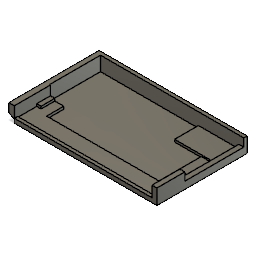
EZ Flash Shell v1 (Autodesk Fusion 360 design; units mm, degrees)
Autodesk Fusion 360 part; units mm, degrees
sketch "Sketch1" plane through (0, 0, 0) normal (0, 1, 0) x (1, 0, 0)
  line L0 (0, 0) -> (53.1, 0)
  line L1 (53.1, 0) -> (53.1, 32)
  line L2 (53.1, 32) -> (0, 32)
  line L3 (0, 32) -> (0, 0)
  line L4 (26.55, 0) -> (26.55, -1.25)
  line L5 (26.55, -1.25) -> (26.55, 33.35)
  line L6 (26.55, 33.35) -> (55, 33.35)
  line L7 (55, 33.35) -> (-1.9, 33.35)
  line L8 (-1.9, 33.35) -> (-1.9, -1.25)
  line L9 (-1.9, -1.25) -> (55, -1.25)
  line L10 (55, -1.25) -> (55, 33.35)
  dimension "d1" = 53.1
  dimension "d2" = 32
  dimension "d3" = 1.25
  dimension "d4" = 34.6
  dimension "d5" = 28.45
  dimension "d6" = 56.9
  dimension "d7" = 34.6
  constraint horizontal L0
  constraint vertical L1
  constraint horizontal L2
  constraint vertical L3
  constraint coincident L0.start L3.end
  constraint midpoint L0 L4.start
  constraint vertical L4
  constraint parallel L4 L5
  constraint perpendicular L5 L6
  constraint horizontal L7
  constraint vertical L8
  constraint horizontal L9
  constraint vertical L10
  measures "d1" distance of L0.start L0.end
  measures "d2" distance of L0.start L2.end
  measures "d3" distance of L4.start L4.end
  measures "d4" distance of L4.end L5.end
  measures "d5" distance of L5.end L6.end
  measures "d6" distance of L6.end L7.end
  measures "d7" distance of L6.end L9.end
extrude "Extrude1" add sketch "Sketch1" along normal blind 1.5
sketch "Sketch2" plane through (0, 1.5, 0) normal (0, 1, 0) x (-1, 0, 0)
  line L0 (-55, 1.25) -> (-55, -33.35)
  line L1 (-55, -33.35) -> (1.9, -33.35)
  line L2 (1.9, -33.35) -> (1.9, 1.25)
  line L3 (1.9, 1.25) -> (-55, 1.25)
  line L4 (1.9, -33.35) -> (-55, -33.35)
  line L5 (-55, -33.35) -> (-55, -32)
  line L6 (-55, -32) -> (1.9, -32)
  line L7 (1.9, -32) -> (1.9, -33.35)
  line L8 (1.9, -32) -> (0, -32)
  line L9 (0, -32) -> (0, 1.25)
  line L10 (0, 1.25) -> (1.9, 1.25)
  line L11 (1.9, 1.25) -> (1.9, -32)
  line L12 (-55, -32) -> (-53.1, -32)
  line L13 (-53.1, -32) -> (-53.1, 1.25)
  line L14 (-53.1, 1.25) -> (-55, 1.25)
  line L15 (-55, 1.25) -> (-55, -32)
  dimension "d10" = 1.35
  dimension "d11" = 1.9
  dimension "d12" = 1.9
  constraint horizontal L4
  constraint vertical L5
  constraint horizontal L6
  constraint vertical L7
  constraint coincident L1.end L2.start
  constraint horizontal L8
  constraint vertical L9
  constraint horizontal L10
  constraint vertical L11
  constraint horizontal L12
  constraint vertical L13
  constraint horizontal L14
  constraint vertical L15
  measures "d10" distance of L1.end L6.end
  measures "d11" distance of L6.end L8.end
  measures "d12" distance of L5.end L12.end
extrude "Extrude2" add sketch "Sketch2" along normal blind 4.4 contours L0 L3 L6 L12 L13 L14 L15 | L0 L1 L2 L4 L5 L6 L7 L8 L12 | L2 L3 L6 L8 L9 L10 L11
sketch "Sketch3" plane through (0, 1.5, 0) normal (0, 1, 0) x (-1, 0, 0)
  line L0 (0, -32) -> (0, 1.25)
  line L1 (0, 1.25) -> (-53.1, 1.25)
  line L2 (-53.1, 1.25) -> (-53.1, -32)
  line L3 (-53.1, -32) -> (0, -32)
  line L4 (0, 1.25) -> (-53.1, 1.25)
  line L5 (-53.1, 1.25) -> (-53.1, 0)
  line L6 (-53.1, 0) -> (0, 0)
  line L7 (0, 0) -> (0, 1.25)
  dimension "d15" = 1.25
  constraint horizontal L4
  constraint vertical L5
  constraint horizontal L6
  constraint vertical L7
  constraint coincident L0.end L1.start
  measures "d15" distance of L0.end L6.end
extrude "Extrude3" add sketch "Sketch3" along normal blind 0.5 contours L0 L1 L2 L4 L5 L6 L7
extrude "Extrude4" add 1 faces at (17.7, 1.5, -21.3333) along direction (0, 1, 0) blind 0.2
sketch "Sketch4" plane through (0, 1.7, 0) normal (0, 1, 0) x (-1, 0, 0)
  line L0 (0, 0) -> (-53.1, 0)
  line L1 (-53.1, 0) -> (-53.1, -32)
  line L2 (-53.1, -32) -> (0, -32)
  line L3 (0, -32) -> (0, 0)
  line L4 (-26.55, 0) -> (-26.55, -6)
  line L5 (-26.55, -32) -> (-26.55, -23)
  line L6 (-53.1, -16) -> (-47.85, -16)
  line L7 (0, -16) -> (-5.25, -16)
  line L8 (-26.55, -6) -> (-5.25, -6)
  line L9 (-26.55, -23) -> (-47.85, -23)
  line L10 (-47.85, -23) -> (-5.25, -23)
  line L11 (-5.25, -23) -> (-5.25, -6)
  line L12 (-5.25, -6) -> (-47.85, -6)
  line L13 (-47.85, -6) -> (-47.85, -23)
  dimension "d20" = 6
  dimension "d21" = 9
  dimension "d22" = 5.25
  dimension "d23" = 5.25
  constraint midpoint L0 L4.start
  constraint perpendicular L0 L4
  constraint midpoint L2 L5.start
  constraint perpendicular L2 L5
  constraint midpoint L1 L6.start
  constraint perpendicular L1 L6
  constraint midpoint L3 L7.start
  constraint perpendicular L3 L7
  constraint perpendicular L4 L8
  constraint perpendicular L5 L9
  constraint horizontal L10
  constraint vertical L11
  constraint horizontal L12
  constraint vertical L13
  measures "d20" distance of L4.start L4.end
  measures "d21" distance of L5.start L5.end
  measures "d22" distance of L6.start L6.end
  measures "d23" distance of L7.start L7.end
extrude "Extrude5" cut sketch "Sketch4" against normal blind 1.3 contours L8 L9 L10 L11 L12 L13
sketch "Sketch5" plane through (0, 1.7, 0) normal (0, 1, 0) x (-1, 0, 0)
  line L0 (-5.25, -23) -> (-47.85, -23)
  line L1 (-47.85, -23) -> (-47.85, -6)
  line L2 (-47.85, -6) -> (-5.25, -6)
  line L3 (-5.25, -6) -> (-5.25, -23)
  line L4 (0, 0) -> (-53.1, 0)
  line L5 (-53.1, 0) -> (-53.1, -32)
  line L6 (-53.1, -32) -> (0, -32)
  line L7 (0, -32) -> (0, 0)
  line L8 (-53.1, 0) -> (-51.1, 0)
  line L9 (-51.1, 0) -> (-51.1, -12.6)
  line L10 (-51.1, -12.6) -> (-53.1, -12.6)
  line L11 (-53.1, -12.6) -> (-53.1, 0)
  line L12 (0, 0) -> (-2, 0)
  line L13 (-2, 0) -> (-2, -12.6)
  line L14 (-2, -12.6) -> (0, -12.6)
  line L15 (0, -12.6) -> (0, 0)
  dimension "d26" = 2
  dimension "d27" = 12.6
  dimension "d28" = 2
  dimension "d29" = 12.6
  constraint horizontal L8
  constraint vertical L9
  constraint horizontal L10
  constraint vertical L11
  constraint coincident L4.end L5.start
  constraint horizontal L12
  constraint vertical L13
  constraint horizontal L14
  constraint vertical L15
  constraint coincident L4.start L7.end
  measures "d26" distance of L4.end L8.end
  measures "d27" distance of L4.end L10.end
  measures "d28" distance of L4.start L12.end
  measures "d29" distance of L4.start L14.end
extrude "Extrude6" add sketch "Sketch5" along normal blind 0.6 contours L4 L7 L12 L13 L14 L15 | L4 L5 L8 L9 L10 L11
sketch "Sketch6" plane through (0, 5.9, 0) normal (0, 1, 0) x (-1, 0, 0)
  line L0 (-53.1, -32) -> (-53.1, 1.25)
  line L1 (-53.1, 1.25) -> (-55, 1.25)
  line L2 (-55, 1.25) -> (-55, -33.35)
  line L3 (-55, -33.35) -> (1.9, -33.35)
  line L4 (1.9, -33.35) -> (1.9, 1.25)
  line L5 (1.9, 1.25) -> (0, 1.25)
  line L6 (0, 1.25) -> (0, -32)
  line L7 (0, -32) -> (-53.1, -32)
  line L8 (-53.1, -32) -> (-55, -32)
  line L9 (-55, -32) -> (-55, -12.5021)
  line L10 (-55, -12.5021) -> (-53.1, -12.5021)
  line L11 (-53.1, -12.5021) -> (-53.1, -32)
  constraint horizontal L8
  constraint vertical L9
  constraint horizontal L10
  constraint vertical L11
  constraint coincident L2 L9.end
  constraint coincident L0.start L7.end
extrude "Extrude7" cut sketch "Sketch6" against normal blind 3.6 contours L0 L2 L8 L9 L10 L11
sketch "Sketch7" plane through (0, 2.3, 0) normal (0, 1, 0) x (-1, 0, 0)
  line L0 (-53.1, -12.6) -> (-51.1, -12.6)
  line L1 (-51.1, -12.6) -> (-51.1, 0)
  line L2 (-51.1, 0) -> (-53.1, 0)
  line L3 (-53.1, 0) -> (-53.1, -12.5021)
  line L4 (-53.1, -12.5021) -> (-55, -12.5021)
  line L5 (-55, -12.5021) -> (-55, -32)
  line L6 (-55, -32) -> (-53.1, -32)
  line L7 (-53.1, -32) -> (-53.1, -12.6)
  line L8 (-51.1, 0) -> (-53.1, 0)
  line L9 (-53.1, 0) -> (-53.1, -6.2511)
  line L10 (-53.1, -6.2511) -> (-51.1, -6.2511)
  line L11 (-51.1, -6.2511) -> (-51.1, 0)
  constraint horizontal L8
  constraint vertical L9
  constraint horizontal L10
  constraint vertical L11
  constraint midpoint L3 L9.end
  constraint coincident L1.end L2.start
extrude "Extrude8" cut sketch "Sketch7" against normal blind 0.6 contours L1 L2 L3 L8 L9 L10 L11
sketch "Sketch8" plane through (0, 2.3, 0) normal (0, 1, 0) x (-1, 0, 0)
  line L0 (0, -12.6) -> (0, 0)
  line L1 (0, 0) -> (-2, 0)
  line L2 (-2, 0) -> (-2, -12.6)
  line L3 (-2, -12.6) -> (0, -12.6)
  line L4 (-2, 0) -> (0, 0)
  line L5 (0, 0) -> (0, -6.3)
  line L6 (0, -6.3) -> (-2, -6.3)
  line L7 (-2, -6.3) -> (-2, 0)
  constraint horizontal L4
  constraint vertical L5
  constraint horizontal L6
  constraint vertical L7
  constraint midpoint L0 L5.end
  constraint coincident L1.end L2.start
extrude "Extrude9" cut sketch "Sketch8" against normal blind 0.6 contours L0 L1 L2 L4 L5 L6 L7
sketch "Sketch9" plane through (0, 1.7, 0) normal (0, 1, 0) x (-1, 0, 0)
  line L0 (-5.25, -23) -> (-47.85, -23)
  line L1 (-47.85, -23) -> (-47.85, -6)
  line L2 (-47.85, -6) -> (-5.25, -6)
  line L3 (-5.25, -6) -> (-5.25, -23)
  line L4 (-51.1, -6.2511) -> (-51.1, -12.6)
  line L5 (-51.1, -12.6) -> (-53.1, -12.6)
  line L6 (-53.1, -12.6) -> (-53.1, -32)
  line L7 (-53.1, -32) -> (0, -32)
  line L8 (0, -32) -> (0, -12.6)
  line L9 (0, -12.6) -> (-2, -12.6)
  line L10 (-2, -12.6) -> (-2, -6.3)
  line L11 (-2, -6.3) -> (0, -6.3)
  line L12 (0, -6.3) -> (0, 0)
  line L13 (0, 0) -> (-53.1, 0)
  line L14 (-53.1, 0) -> (-53.1, -6.2511)
  line L15 (-53.1, -6.2511) -> (-51.1, -6.2511)
  line L16 (0, -12.6) -> (-53.1, -12.6)
  line L17 (-53.1, -12.6) -> (-53.1, -32)
  line L18 (-53.1, -32) -> (0, -32)
  line L19 (0, -32) -> (0, -12.6)
  constraint horizontal L16
  constraint vertical L17
  constraint horizontal L18
  constraint vertical L19
  constraint coincident L6.end L7.start
  constraint coincident L8.end L9.start
extrude "Extrude10" cut sketch "Sketch9" against normal blind 1 contours L0 L1 L3 L5 L6 L7 L8 L9 L16 L17 L18 L19
sketch "Sketch10" plane through (0, 1.7, 0) normal (0, 1, 0) x (-1, 0, 0)
  line L0 (-5.25, -12.6) -> (-2, -12.6)
  line L1 (-2, -12.6) -> (-2, -6.3)
  line L2 (-2, -6.3) -> (0, -6.3)
  line L3 (0, -6.3) -> (0, 0)
  line L4 (0, 0) -> (-53.1, 0)
  line L5 (-53.1, 0) -> (-53.1, -6.2511)
  line L6 (-53.1, -6.2511) -> (-51.1, -6.2511)
  line L7 (-51.1, -6.2511) -> (-51.1, -12.6)
  line L8 (-51.1, -12.6) -> (-47.85, -12.6)
  line L9 (-47.85, -12.6) -> (-47.85, -6)
  line L10 (-47.85, -6) -> (-5.25, -6)
  line L11 (-5.25, -6) -> (-5.25, -12.6)
  line L12 (-47.85, -6) -> (-51.1, -6)
  line L13 (-51.1, -6) -> (-51.1, -12.6)
  line L14 (-51.1, -12.6) -> (-47.85, -12.6)
  line L15 (-47.85, -12.6) -> (-47.85, -6)
  constraint horizontal L12
  constraint vertical L13
  constraint horizontal L14
  constraint vertical L15
  constraint coincident L7.end L8.start
  constraint coincident L9.end L10.start
extrude "Extrude11" cut sketch "Sketch10" against normal blind 1 contours L7 L8 L9 L12 L13 L14 L15
sketch "Sketch11" plane through (0, 0.7, 0) normal (0, 1, 0) x (-1, 0, 0)
  line L0 (0, -32) -> (0, -12.6)
  line L1 (0, -12.6) -> (-5.25, -12.6)
  line L2 (-5.25, -12.6) -> (-5.25, -23)
  line L3 (-5.25, -23) -> (-47.85, -23)
  line L4 (-47.85, -23) -> (-47.85, -6)
  line L5 (-47.85, -6) -> (-51.1, -6)
  line L6 (-51.1, -6) -> (-51.1, -12.6)
  line L7 (-51.1, -12.6) -> (-53.1, -12.6)
  line L8 (-53.1, -12.6) -> (-53.1, -32)
  line L9 (-53.1, -32) -> (0, -32)
  line L10 (-26.55, -32) -> (-53.1, -32)
  line L11 (-53.1, -32) -> (-53.1, -23)
  line L12 (-53.1, -23) -> (-26.55, -23)
  line L13 (-26.55, -23) -> (-26.55, -32)
  constraint horizontal L10
  constraint vertical L11
  constraint horizontal L12
  constraint vertical L13
  constraint coincident L8 L11.end
  constraint midpoint L9 L10.start
extrude "Extrude12" add sketch "Sketch11" along normal blind 1 contours L3 L8 L9 L10 L11 L12 L13
extrude "Extrude13" cut 1 faces at (26.55, 1.0333, -26) along direction (1, 0, 0) blind 11
extrude "Extrude14" cut 1 faces at (54.3667, 4.7, -12.5021) along direction (0, 0, 1) blind 3
extrude "Extrude15" add 1 faces at (53.1, 4.7, -4.8344) along direction (-1, 0, 0) blind 0.5
sketch "Sketch12" plane through (0, 0, 0) normal (1, 0, 0) x (0, 0, -1)
  line L0 (6.3, 2.3) -> (12.6, 2.3)
  line L1 (12.6, 2.3) -> (12.6, 0.7)
  line L2 (12.6, 0.7) -> (32, 0.7)
  line L3 (32, 0.7) -> (32, 5.9)
  line L4 (32, 5.9) -> (-1.25, 5.9)
  line L5 (-1.25, 5.9) -> (-1.25, 2)
  line L6 (-1.25, 2) -> (0, 2)
  line L7 (0, 2) -> (0, 1.7)
  line L8 (0, 1.7) -> (6.3, 1.7)
  line L9 (6.3, 1.7) -> (6.3, 2.3)
  line L10 (-1.25, 5.9) -> (12.6, 5.9)
  line L11 (12.6, 5.9) -> (12.6, -0.6915)
  line L12 (12.6, -0.6915) -> (-1.25, -0.6915)
  line L13 (-1.25, -0.6915) -> (-1.25, 5.9)
  dimension "d50" = 13.85
  constraint horizontal L10
  constraint vertical L11
  constraint horizontal L12
  constraint vertical L13
  constraint coincident L4.end L5.start
  measures "d50" distance of L4.end L10.end
extrude "Extrude16" add sketch "Sketch12" along normal blind 0.5 contours L0 L4 L5 L6 L7 L8 L9 L10 L11 L13
sketch "Sketch13" plane through (0, 0, 1.25) normal (0, 0, 1) x (1, 0, 0)
  line L0 (-1.9, 0) -> (55, 0)
  line L1 (55, 0) -> (55, 5.9)
  line L2 (55, 5.9) -> (52.6, 5.9)
  line L3 (52.6, 5.9) -> (52.6, 2)
  line L4 (52.6, 2) -> (0.5, 2)
  line L5 (0.5, 2) -> (0.5, 5.9)
  line L6 (0.5, 5.9) -> (-1.9, 5.9)
  line L7 (-1.9, 5.9) -> (-1.9, 0)
  line L8 (55, 0) -> (53, 0)
  line L9 (53, 0) -> (53, 2.3)
  line L10 (53, 2.3) -> (55, 2.3)
  line L11 (55, 2.3) -> (55, 0)
  line L12 (-1.9, 0) -> (0.1, 0)
  line L13 (0.1, 0) -> (0.1, 2.3)
  line L14 (0.1, 2.3) -> (-1.9, 2.3)
  line L15 (-1.9, 2.3) -> (-1.9, 0)
  dimension "d53" = 2
  dimension "d54" = 2.3
  dimension "d55" = 2
  dimension "d56" = 2.3
  constraint horizontal L8
  constraint vertical L9
  constraint horizontal L10
  constraint vertical L11
  constraint coincident L0.end L1.start
  constraint horizontal L12
  constraint vertical L13
  constraint horizontal L14
  constraint vertical L15
  constraint coincident L0.start L7.end
  measures "d53" distance of L0.end L8.end
  measures "d54" distance of L0.end L10.end
  measures "d55" distance of L0.start L12.end
  measures "d56" distance of L0.start L14.end
extrude "Extrude17" cut sketch "Sketch13" against normal blind 12 contours L0 L7 L12 L13 L14 L15 | L0 L1 L8 L9 L10 L11
sketch "Sketch14" plane through (0, 2.3, 0) normal (0, 1, 0) x (-1, 0, 0)
  line L0 (-53, -9.5021) -> (-53, -10.75)
  line L1 (-53, -10.75) -> (-55, -10.75)
  line L2 (-55, -10.75) -> (-55, -32)
  line L3 (-55, -32) -> (-53.1, -32)
  line L4 (-53.1, -32) -> (-53.1, -12.6)
  line L5 (-53.1, -12.6) -> (-51.1, -12.6)
  line L6 (-51.1, -12.6) -> (-51.1, -6.2511)
  line L7 (-51.1, -6.2511) -> (-52.6, -6.2511)
  line L8 (-52.6, -6.2511) -> (-52.6, -9.5021)
  line L9 (-52.6, -9.5021) -> (-53, -9.5021)
  line L10 (-51.1, -9.4255) -> (-55, -9.4255)
  line L11 (-55, -9.4255) -> (-55, -32)
  line L12 (-55, -32) -> (-51.1, -32)
  line L13 (-51.1, -32) -> (-51.1, -9.4255)
  constraint horizontal L10
  constraint vertical L11
  constraint horizontal L12
  constraint vertical L13
  constraint coincident L2.end L3.start
  constraint midpoint L6 L10.start
extrude "Extrude18" add sketch "Sketch14" along normal blind 0.5 contours L0 L1 L2 L3 L4 L5 L6 L8 L9 L10 L11 L12 L13 | L0 L1 L8 L9 L10 L11
extrude "Extrude19" add 1 faces at (53, 0.7667, -2.75) along direction (1, 0, 0) blind 0.5
extrude "Extrude20" add 1 faces at (0.1, 0.7667, -2.75) along direction (-1, 0, 0) blind 0.5
extrude "Extrude21" cut 1 faces at (54.3667, 2.8, -18.034) along direction (0, -1, 0) blind 0.5
extrude "Extrude22" add 1 faces at (54, 2.3, -5.9181) along direction (0, -1, 0) blind 0.4
sketch "Sketch15" plane through (0, 0, -9.5021) normal (0, 0, -1) x (-1, 0, 0)
  line L0 (-52.6, 2.3) -> (-52.6, 5.9)
  line L1 (-52.6, 5.9) -> (-55, 5.9)
  line L2 (-55, 5.9) -> (-55, 1.9)
  line L3 (-55, 1.9) -> (-53.5, 1.9)
  line L4 (-53.5, 1.9) -> (-53.5, 2.3)
  line L5 (-53.5, 2.3) -> (-52.6, 2.3)
  line L6 (-53.5, 2.3) -> (-55, 2.3)
  line L7 (-55, 2.3) -> (-55, 1.9)
  line L8 (-55, 1.9) -> (-53.5, 1.9)
  line L9 (-53.5, 1.9) -> (-53.5, 2.3)
  constraint horizontal L6
  constraint vertical L7
  constraint horizontal L8
  constraint vertical L9
  constraint coincident L2.end L3.start
  constraint coincident L4.end L5.start
extrude "Extrude23" add sketch "Sketch15" along normal blind 1.248 contours L2 L3 L4 L6 L7 L8 L9
extrude "Extrude24" add 1 faces at (-0.9, 2.3, -2.75) along direction (0, -1, 0) blind 0.4
extrude "Extrude25" cut 1 faces at (0.5, 4.7, -5.8833) along direction (-1, 0, 0) blind 0.5
extrude "Extrude26" cut 1 faces at (52.6, 4.7, -4.8344) along direction (1, 0, 0) blind 0.5
move_face "MoveFace1" by (-0.2, 0, 0) 4 faces at (0, 2.9667, -25.5333) (-0.4, 0.6333, -2.75) (-1.9, 2.6, -25.8167) (2, 1.9, -8.4)
chamfer "Chamfer1" distance 0.5 angle 45 1 edges at (-0.6, 1.9, -4.75)
chamfer "Chamfer2" distance 0.5 angle 45 1 edges at (-2.1, 1.9, -4.75)
chamfer "Chamfer3" distance 0.5 angle 45 1 edges at (53.5, 1.9, -4.75)
sketch "Sketch16" plane through (0, 2.3, 0) normal (0, 1, 0) x (-1, 0, 0)
  line L0 (-55, -9.5021) -> (-55, -32)
  line L1 (-55, -32) -> (-53.1, -32)
  line L2 (-53.1, -32) -> (-53.1, -12.6)
  line L3 (-53.1, -12.6) -> (-51.1, -12.6)
  line L4 (-51.1, -12.6) -> (-51.1, -6.2511)
  line L5 (-51.1, -6.2511) -> (-53.1, -6.2511)
  line L6 (-53.1, -6.2511) -> (-53.1, -9.5021)
  line L7 (-53.1, -9.5021) -> (-55, -9.5021)
  line L8 (-55, -9.5021) -> (-53.1, -9.5021)
  line L9 (-53.1, -9.5021) -> (-53.1, -32)
  line L10 (-53.1, -32) -> (-55, -32)
  line L11 (-55, -32) -> (-55, -9.5021)
  constraint horizontal L8
  constraint vertical L9
  constraint horizontal L10
  constraint vertical L11
  constraint coincident L1.end L2.start
  constraint coincident L0.start L7.end
extrude "Extrude27" add sketch "Sketch16" along normal blind 0.5 contours L0 L1 L2 L7 L8 L9 L10 L11
chamfer "Chamfer4" distance 0.5 angle 45 1 edges at (55, 1.9, -4.75)
extrude "Extrude28" cut 2 faces at (19.3833, 1.7, -2) (47.9167, 1.7, -26) along direction (0, -1, 0) blind 0.4
extrude "Extrude29" cut 1 faces at (17.5667, 2, 0.8333) along direction (0, -1, 0) blind 0.3
extrude "Extrude30" cut 1 faces at (14.2, 0.7, -29) along direction (0, -1, 0) blind 0.3
move_face "MoveFace2" by (0, 0, -0.2) 2 faces at (12.3833, 2.5333, -32) (16.9333, 1.9667, -33.35)
sketch "Sketch17" plane through (-0.2, 0, 0) normal (1, 0, 0) x (0, 0, -1)
  line L0 (12.6, 2.3) -> (12.6, 0.4)
  line L1 (12.6, 0.4) -> (32.2, 0.4)
  line L2 (32.2, 0.4) -> (32.2, 5.9)
  line L3 (32.2, 5.9) -> (-1.25, 5.9)
  line L4 (-1.25, 5.9) -> (-1.25, 1.7)
  line L5 (-1.25, 1.7) -> (0, 1.7)
  line L6 (0, 1.7) -> (0, 1.3)
  line L7 (0, 1.3) -> (6.3, 1.3)
  line L8 (6.3, 1.3) -> (6.3, 2.3)
  line L9 (6.3, 2.3) -> (12.6, 2.3)
  line L10 (12.6, 2.3) -> (-1.25, 2.3)
  line L11 (-1.25, 2.3) -> (-1.25, 5.9)
  line L12 (-1.25, 5.9) -> (12.6, 5.9)
  line L13 (12.6, 5.9) -> (12.6, 2.3)
  constraint horizontal L10
  constraint vertical L11
  constraint horizontal L12
  constraint vertical L13
  constraint coincident L3.end L4.start
  constraint coincident L0.start L9.end
extrude "Extrude31" add sketch "Sketch17" along normal blind 0.8 contours L3 L4 L9 L10 L11 L12 L13 | L4 L5 L6 L7 L8 L10
sketch "Sketch18" plane through (0, 0, 1.25) normal (0, 0, 1) x (1, 0, 0)
  line L0 (53.1, 5.9) -> (53.1, 1.7)
  line L1 (53.1, 1.7) -> (0.6, 1.7)
  line L2 (0.6, 1.7) -> (0.6, 5.9)
  line L3 (0.6, 5.9) -> (-2.1, 5.9)
  line L4 (-2.1, 5.9) -> (-2.1, 2.4)
  line L5 (-2.1, 2.4) -> (-1.6, 1.9)
  line L6 (-1.6, 1.9) -> (-1.1, 1.9)
  line L7 (-1.1, 1.9) -> (-0.6, 1.4)
  line L8 (-0.6, 1.4) -> (-0.6, 0)
  line L9 (-0.6, 0) -> (53.5, 0)
  line L10 (53.5, 0) -> (53.5, 1.4)
  line L11 (53.5, 1.4) -> (54, 1.9)
  line L12 (54, 1.9) -> (54.5, 1.9)
  line L13 (54.5, 1.9) -> (55, 2.4)
  line L14 (55, 2.4) -> (55, 5.9)
  line L15 (55, 5.9) -> (53.1, 5.9)
  line L16 (-2.1, 2.4) -> (-0.1, 2.4)
  line L17 (-0.1, 2.4) -> (-0.1, 0)
  line L18 (-0.1, 0) -> (-2.1, 0)
  line L19 (-2.1, 0) -> (-2.1, 2.4)
  dimension "d91" = 2
  constraint horizontal L16
  constraint vertical L17
  constraint horizontal L18
  constraint vertical L19
  constraint coincident L4.end L5.start
  measures "d91" distance of L4.end L16.end
extrude "Extrude32" cut sketch "Sketch18" against normal blind 12 contours L5 L6 L7 L8 L9 L16 L17 L18
sketch "Sketch19" plane through (0, 0, 1.25) normal (0, 0, 1) x (1, 0, 0)
  line L0 (-0.1, 2.4) -> (-0.1, 0)
  line L1 (-0.1, 0) -> (53.5, 0)
  line L2 (53.5, 0) -> (53.5, 1.4)
  line L3 (53.5, 1.4) -> (54, 1.9)
  line L4 (54, 1.9) -> (54.5, 1.9)
  line L5 (54.5, 1.9) -> (55, 2.4)
  line L6 (55, 2.4) -> (55, 5.9)
  line L7 (55, 5.9) -> (53.1, 5.9)
  line L8 (53.1, 5.9) -> (53.1, 1.7)
  line L9 (53.1, 1.7) -> (0.6, 1.7)
  line L10 (0.6, 1.7) -> (0.6, 5.9)
  line L11 (0.6, 5.9) -> (-2.1, 5.9)
  line L12 (-2.1, 5.9) -> (-2.1, 2.4)
  line L13 (-2.1, 2.4) -> (-0.1, 2.4)
  line L14 (53.5, 0) -> (55, 0)
  line L15 (55, 0) -> (55, 2.4)
  line L16 (55, 2.4) -> (53.5, 2.4)
  line L17 (53.5, 2.4) -> (53.5, 0)
  constraint horizontal L14
  constraint vertical L15
  constraint horizontal L16
  constraint vertical L17
  constraint coincident L5.end L6.start
  constraint coincident L1.end L2.start
extrude "Extrude33" add sketch "Sketch19" against normal blind 12 contours L2 L3 L4 L5 L14 L15 L17
chamfer "Chamfer5" distance 1 distance2 2 1 edges at (-0.1, 2.4, -4.75) measured on face at (-0.1, 1.6, -2.75)
extrude "Extrude34" cut 1 faces at (0.6, 4.7, -5.8833) along direction (-1, 0, 0) blind 0.5
extrude "Extrude35" cut 1 faces at (51.7667, 1.9667, -6.2511) along direction (0, 0, -1) blind 0.049
extrude "Extrude36" cut 1 faces at (1.2333, 1.6333, -6.3) along direction (0, 0, -1) blind 0.0001
extrude "Extrude37" cut 2 faces at (51.7667, 1.9667, -6.3001) (1.2333, 1.6333, -6.3001) along direction (0, 0, -1) blind 1
extrude "Extrude38" add 1 faces at (19.4833, 1.3, -2) along direction (0, 1, 0) blind 0.1
equation "d5 = ( 56.9 / 2 ) * 1 mm"
equation "d85 = -0.70 mm + 0.4 mm"
equation "d102 = -6.104E-05 mm"
